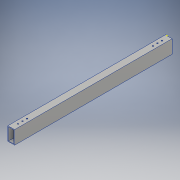
# Autodesk Inventor part: nhk9
Saved by Autodesk Inventor 2019 (Build 230136000, 136)
## iProperties
Created: 2022-02-15
Part Number: nhk9
Material: アルミニウム 6061
Document SubType Name: Modeling
Designer: yuta
Density: 2.7 g/cm^3
Appearance: アルミニウム - フラット
Author: yuta
Autodesk Inventor part; units mm, degrees
ref_plane "YZ Plane" through (0, 0, 0) normal (1, 0, 0) x (0, 1, 0)
ref_plane "XZ Plane" through (0, 0, 0) normal (0, 1, 0) x (-1, 0, 0)
ref_plane "XY Plane" through (0, 0, 0) normal (0, 0, 1) x (1, 0, 0)
sketch "スケッチ1" plane through (0, 0, 0) normal (0, 0, 1) x (1, 0, 0)
  line L0 (-3.8522, 2.7979) -> (11.1478, 2.7979)
  line L1 (11.1478, 2.7979) -> (11.1478, -27.2021)
  line L2 (11.1478, -27.2021) -> (-3.8522, -27.2021)
  line L3 (-3.8522, -27.2021) -> (-3.8522, 2.7979)
  point P0 (0, 0)
  dimension "d0" = 15
  dimension "d1" = 30
  constraints: 8 end point, 2 parallel, 1 horizontal, 1 perpendicular
  measures "d0" distance of L1.end L2.end
  measures "d1" distance of L0.end L1.end
extrude "押し出し1" add sketch "スケッチ1" along normal blind 350
sketch "スケッチ2" plane through (-3.8522, 2.7979, 0) normal (0, 1, 0) x (1, 0, 0)
  circle A0 centre (7.5, -335) radius 1.5
  line L0 (15, -350) -> (0, -350) projected
  circle A1 centre (7.5, -325) radius 1.5
  circle A2 centre (7.5, -315) radius 1.5
  line L1 (0, 0) -> (0, -350) projected
  line L2 (15, 0) -> (15, -350) projected
  circle A3 centre (7.5, -15) radius 1.5
  line L3 (0, 0) -> (15, 0) projected
  circle A4 centre (7.5, -25) radius 1.5
  circle A5 centre (7.5, -35) radius 1.5
  point P0 (3.8522, 0)
  dimension "d4" = 3
  dimension "d5" = 15
  dimension "d6" = 3
  dimension "d7" = 3
  dimension "d8" = 10
  dimension "d9" = 10
  dimension "d10" = 7.5
  dimension "d11" = 7.5
  dimension "d12" = 7.5
  dimension "d13" = 3
  dimension "d14" = 15
  dimension "d15" = 7.5
  dimension "d16" = 3
  dimension "d17" = 3
  dimension "d18" = 10
  dimension "d19" = 10
  constraints: 6 centre point
  measures "d4" diameter of A0
  measures "d5" distance from line of A0.centre L0
  measures "d6" diameter of A1
  measures "d7" diameter of A2
  measures "d8" distance of A1.centre A0.centre
  measures "d9" distance of A2.centre A1.centre
  measures "d10" distance from line of L1 A0.centre
  measures "d11" distance from line of L2 A1.centre
  measures "d12" distance from line of L1 A2.centre
  measures "d13" diameter of A3
  measures "d14" distance from line of L3 A3.centre
  measures "d15" distance from line of L2 A3.centre
  measures "d16" diameter of A4
  measures "d17" diameter of A5
  measures "d18" distance of A4.centre A3.centre
  measures "d19" distance of A4.centre A5.centre
hole "穴1" at (3.6478, 2.7979, 335) at (3.6478, 2.7979, 325) at (3.6478, 2.7979, 315) at (3.6478, 2.7979, 35) at (3.6478, 2.7979, 25) at (3.6478, 2.7979, 15) direction (0, -1, 0) diameter 3 depth 30
sketch "スケッチ3" plane through (0, 0, 0) normal (0, 0, -1) x (-1, 0, 0)
  line L0 (-9.6478, 1.2979) -> (2.3522, 1.2979)
  line L1 (2.3522, 1.2979) -> (2.3522, -25.7021)
  line L2 (2.3522, -25.7021) -> (-9.6478, -25.7021)
  line L3 (-9.6478, -25.7021) -> (-9.6478, 1.2979)
  line L4 (3.8522, 2.7979) -> (-11.1478, 2.7979) projected
  line L5 (-11.1478, 2.7979) -> (-11.1478, -27.2021) projected
  point P0 (0, 0)
  dimension "d27" = 12
  dimension "d28" = 27
  dimension "d29" = 1.5
  dimension "d30" = 1.5
  constraints: 8 end point, 2 parallel, 1 horizontal, 1 perpendicular
  measures "d27" distance of L1.end L2.end
  measures "d28" distance of L0.end L1.end
  measures "d29" distance between parallel lines of L0 L4
  measures "d30" distance between parallel lines of L5 L3
extrude "押し出し2" cut sketch "スケッチ3" against normal blind 350
sketch "スケッチ4" plane through (-3.8522, 2.7979, 0) normal (0, 1, 0) x (1, 0, 0)
  point P0 (3.8522, 0)
